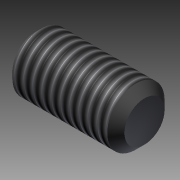
# Autodesk Inventor part: SET-SCREW5-9.5
Saved by Autodesk Inventor 2016 (Build 200138000, 138)
## iProperties
Category: PARTsolutions
Company: MISUMI
Created: 2016-11-09
Part Number: SET-SCREW5-9.5
Catalog Web Link: www.cadenas.de
Description: SET-SCREW-Set Screw - Flat End
Vendor: MISUMI
Document SubType Name: Modeling
Designer: psAdmin
Manufacturer: MISUMI
Mass: 0.168784 g
Surface Area: 1.94116 cm^2
Volume: 0.168784 cm^3
Density: 1 g/cm^3
Material: 一般
Appearance: PSOLRGB-192-192-192
PSOL_IDENT_0: {$CADENAS_DATA\23d-libs\misumi\metric\accessories\set_screw.prj},174 {VTYP=3D},{NB=SET-SCREW5-9.5},{
PSOL_IDENT_1: LINA=SET-SCREW5-9.5},{NN=SET-SCREW},{DATE=17.06.2016 05:56:50},{GEOMDATE=11.12.2013 00:00:00},{VERSI
PSOL_IDENT_2: ON=},{LINEID=80},{LINESUBID=-1},{WBVAR=L}  {NB=SET-SCREW5-9.5},{LINA=SET-SCREW5-9.5},{KT=DUMMY},{PN=
PSOL_IDENT_3: SET-SCREW5-9.5},{TYPE=SET-SCREW},{M=5.0},{P=0.80},{L=9.5},{LMIN=2.8},{LALG=[2.8:42/0.1]},{B=2.5},{C=
PSOL_IDENT_4: 2.0},{DD=3.5}
NN: SET-SCREW
NT: Set Screw - Flat End
NB: SET-SCREW5-9.5
NBSYN: $PN.
LINA: SET-SCREW5-9.5
PN: SET-SCREW5-9.5
M: 5.0
P: 0.80
L: 9.5
B: 2.5
C: 2.0
DD: 3.5
SUPPLIER: MISUMI
ARTICLENO: SET-SCREW5-9.5
BOMINFO: SET-SCREW5-9.5
CREATOR: CADENAS GmbH
Title: SET-SCREW5-9.5
Author: Cadenas PARTsolutions
Comments: Set Screw - Flat End
Autodesk Inventor part; units mm, degrees
sketch "Sketch_1" plane through (0, 0, 0) normal (0, 0, 1) x (1, 0, 0)
  line L0 (0, 0) -> (-9.5, 0)
  line L1 (-9.5, 0) -> (-9.5, 2.0095)
  line L2 (-9.5, 2.0095) -> (-9.0095, 2.5)
  line L3 (-9.0095, 2.5) -> (-0.75, 2.5)
  line L4 (-0.75, 2.5) -> (0, 1.75)
  line L5 (0, 1.75) -> (0, 0)
  line L6 (0, 0) -> (-9.5, 0)
  constraints: 14 end point
revolve "Revolution1" add sketch "Sketch_1" angle 360 about axis through (0, 0, 0) along (1, 0, 0)
thread "Thread1" size "M5x0.8" class "6g" standard "ISO Metric profile" full length
sketch "Sketch_2" plane through (-9.5, 0, 0) normal (-1, 0, 0) x (0, 1, 0)
  line L0 (-1.25, 0.7217) -> (-1.25, -0.7217)
  line L1 (-1.25, -0.7217) -> (0, -1.4434)
  line L2 (0, -1.4434) -> (1.25, -0.7217)
  line L3 (1.25, -0.7217) -> (1.25, 0.7217)
  line L4 (1.25, 0.7217) -> (0, 1.4434)
  line L5 (0, 1.4434) -> (-1.25, 0.7217)
  constraints: 12 end point
extrude "Extrusion1" cut sketch "Sketch_2" against normal blind 2
sketch "Sketch_3" plane through (0, 0, 0) normal (0, 0, 1) x (1, 0, 0)
  line L0 (-6.7783, 0) -> (-7.5, 0)
  line L1 (-7.5, 0) -> (-7.5, 1.25)
  line L2 (-7.5, 1.25) -> (-6.7783, 0)
  line L3 (-6.7783, 0) -> (-7.5, 0)
  constraints: 8 end point
revolve "Revolution2" cut sketch "Sketch_3" angle 360 about axis through (-6.7783, 0, 0) along (1, 0, 0)
ref_plane "CP_XY" through (0, 0, 0) normal (1, 0, 0) x (0, 0, -1)
ref_plane "CP_YZ" through (0, 0, 0) normal (0, 0, -1) x (0, 1, 0)
ref_plane "CP_ZX" through (0, 0, 0) normal (0, 1, 0) x (1, 0, 0)
body "Solid1"
